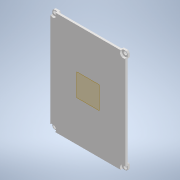
# Autodesk Inventor part: Bottom_lid
Saved by Autodesk Inventor 2022 (Build 260153000, 153)
## iProperties
Created: 2021-01-26
Part Number: Bottom_lid
Material: Generic
Document SubType Name: Modeling
Designer: simen
Density: 1 g/cm^3
Appearance: Default
Author: simen
## iProperties of the stored document Bottom_lid_3DPrint.ipt
Created: 2021-12-09
Part Number: Bottom_lid_3DPrint
Material: Generic
Document SubType Name: Modeling
Designer: simen
Density: 1 g/cm^3
Appearance: Default
Author: simen
Autodesk Inventor part; units mm, degrees
ref_plane "YZ Plane" through (0, 0, 0) normal (1, 0, 0) x (0, 1, 0)
ref_plane "XZ Plane" through (0, 0, 0) normal (0, 1, 0) x (-1, 0, 0)
ref_plane "XY Plane" through (0, 0, 0) normal (0, 0, 1) x (1, 0, 0)
ref_plane "Work Plane3" through (0, 0, 0) normal (0, 0, 1) x (1, 0, 0)
sketch "Sketch1" plane through (0, 0, 0) normal (0, 0, 1) x (1, 0, 0)
  line L0 (37, 49) -> (37, -49) projected
  arc A0 (37, 49) -> (35, 51) centre (35, 49) ccw projected
  line L1 (-35, 51) -> (35, 51) projected
  line L2 (-37, -49) -> (-37, 49) projected
  arc A1 (-35, 51) -> (-37, 49) centre (-35, 49) ccw projected
  arc A2 (-37, -49) -> (-35, -51) centre (-35, -49) ccw projected
  line L3 (35, -51) -> (-35, -51) projected
  arc A3 (35, -51) -> (37, -49) centre (35, -49) ccw projected
  arc A4 (36.8, 49) -> (35, 50.8) centre (35, 49) ccw
  line L4 (36.8, 49) -> (36.8, -49)
  arc A5 (35, -50.8) -> (36.8, -49) centre (35, -49) ccw
  line L5 (35, -50.8) -> (-35, -50.8)
  arc A6 (-36.8, -49) -> (-35, -50.8) centre (-35, -49) ccw
  line L6 (-36.8, -49) -> (-36.8, 49)
  arc A7 (-35, 50.8) -> (-36.8, 49) centre (-35, 49) ccw
  line L7 (-35, 50.8) -> (35, 50.8)
  circle A8 centre (34.6, 48.6) radius 1.6
  circle A9 centre (34.6, -48.6) radius 1.6
  circle A10 centre (-34.6, -48.6) radius 1.6
  circle A11 centre (-34.6, 48.6) radius 1.6
  point P0 (0, 0)
  point P1 (-33, 42)
  dimension "d0" = 0.2
  dimension "d1" = 3.2
  dimension "d2" = 3.2
  dimension "d3" = 3.2
  dimension "d11" = 3.2
  dimension "d34" = 2.2
  dimension "d35" = 2.2
  dimension "d36" = 2.2
  dimension "d37" = 2.2
  dimension "d39" = 2.2
  dimension "d40" = 2.2
  dimension "d41" = 2.2
  dimension "d42" = 2.2
  constraints: 8 centre point, 8 end point, 8 point on circle, 1 coincident, 7 other
  measures "d0" distance between parallel lines of L1 L7
  measures "d1" diameter of A8
  measures "d2" diameter of A9
  measures "d3" diameter of A10
  measures "d11" diameter of A11
  measures "d34" distance from line of L5 A9.centre
  measures "d35" distance from line of L4 A9.centre
  measures "d36" distance from line of L4 A8.centre
  measures "d37" distance from line of L7 A8.centre
  measures "d39" distance from line of L7 A11.centre
  measures "d40" distance from line of L6 A11.centre
  measures "d41" distance from line of L6 A10.centre
  measures "d42" distance from line of L5 A10.centre
extrude "Extrusion1" add sketch "Sketch1" against normal blind 2 contours L4 A5 L5 A6 L6 A7 L7 A4
sketch "Sketch3" plane through (0, 0, -2) normal (0, 0, -1) x (-1, 0, 0)
  circle A0 centre (34.6, 48.6) radius 1.6 projected
  circle A1 centre (34.6, -48.6) radius 1.6 projected
  circle A2 centre (-34.6, -48.6) radius 1.6 projected
  arc A3 (-36.8, -49) -> (-35, -50.8) centre (-35, -49) ccw projected
  line L0 (-36.8, 49) -> (-36.8, -49) projected
  line L1 (-35, -50.8) -> (35, -50.8) projected
  arc A4 (-35, 50.8) -> (-36.8, 49) centre (-35, 49) ccw projected
  line L2 (35, 50.8) -> (-35, 50.8) projected
  arc A5 (36.8, 49) -> (35, 50.8) centre (35, 49) ccw projected
  line L3 (36.8, -49) -> (36.8, 49) projected
  arc A6 (35, -50.8) -> (36.8, -49) centre (35, -49) ccw projected
  circle A7 centre (34.6, -48.6) radius 4
  circle A8 centre (-34.6, 48.6) radius 1.6 projected
  circle A9 centre (-34.6, 48.6) radius 4
  circle A10 centre (-34.6, -48.6) radius 4
  circle A11 centre (34.6, 48.6) radius 4
  point P0 (0, 0)
  point P1 (36.8, -45.2593)
  point P2 (31.2593, -50.8)
  point P3 (-36.8, 45.2593)
  point P4 (-31.2593, 50.8)
  point P5 (-31.2593, -50.8)
  point P6 (-36.8, -45.2593)
  point P7 (31.2593, 50.8)
  point P8 (36.8, 45.2593)
  dimension "d28" = 8
  dimension "d29" = 8
  dimension "d30" = 8
  dimension "d32" = 8
  constraints: 4 centre point, 4 coincident
  measures "d28" diameter of A9
  measures "d29" diameter of A10
  measures "d30" diameter of A7
  measures "d32" diameter of A11
extrude "Extrusion2" add sketch "Sketch3" along normal blind 2 contours L0 A10 L1 A3 | L0 A4 L2 A9 | A7 L3 A6 L1 | L2 A5 L3 A11 picked at (-36.5389, -47.3719) picked at (-36.5389, 47.3719) picked at (36.5389, -47.3719) picked at (36.5389, 47.3719)
sketch "Sketch4" plane through (0, 0, 0) normal (0, 0, 1) x (1, 0, 0)
  line L0 (36.8, -49) -> (36.8, 49) projected
  arc A0 (36.8, 49) -> (35, 50.8) centre (35, 49) ccw projected
  line L1 (35, 50.8) -> (-35, 50.8) projected
  arc A1 (-35, 50.8) -> (-36.8, 49) centre (-35, 49) ccw projected
  line L2 (-36.8, 49) -> (-36.8, -49) projected
  arc A2 (-36.8, -49) -> (-35, -50.8) centre (-35, -49) ccw projected
  line L3 (-35, -50.8) -> (35, -50.8) projected
  arc A3 (35, -50.8) -> (36.8, -49) centre (35, -49) ccw projected
  circle A4 centre (-34.6, 48.6) radius 1.6 projected
  circle A5 centre (-34.6, -48.6) radius 1.6 projected
  circle A6 centre (34.6, -48.6) radius 1.6 projected
  circle A7 centre (34.6, 48.6) radius 3.25
  circle A8 centre (34.6, -48.6) radius 1.6 projected
  circle A9 centre (34.6, -48.6) radius 3.25
  circle A10 centre (-34.6, -48.6) radius 1.6 projected
  circle A11 centre (-34.6, -48.6) radius 3.25
  circle A12 centre (-34.6, 48.6) radius 3.25
  point P0 (0, 0)
  dimension "d22" = 6.5
  dimension "d23" = 6.5
  dimension "d24" = 6.5
  dimension "d25" = 6.5
  constraints: 4 centre point, 3 coincident
  measures "d22" diameter of A7
  measures "d23" diameter of A9
  measures "d24" diameter of A11
  measures "d25" diameter of A12
extrude "Extrusion3" cut sketch "Sketch4" against normal blind 2 contours A3 L3 A9 L0 | L0 A9 L3 A3 | A7 L1 A0 L0 | L0 A0 L1 A7 | A11 L2 A2 L3 | L3 A2 L2 A11 | A12 L2 A1 L1 | L1 A1 L2 A12
fillet "Fillet1" radius 1.5 4 edges at (31.7716, -45.7716, -2) (31.7716, 45.7716, -2) (-31.7716, 45.7716, -2) (-31.7716, -45.7716, -2)
body "Solid1"
